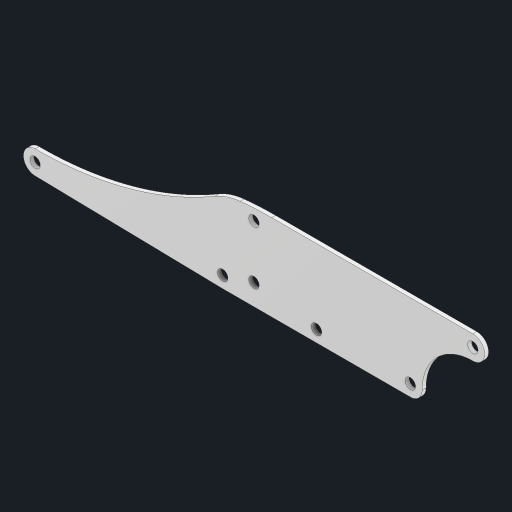
# Autodesk Inventor part: intake_base
Saved by Autodesk Inventor 2024 (Build 280153000, 153)
## iProperties
Created: 2023-08-21
Part Number: intake_base
Material: Acetal Resin, White
Document SubType Name: Modeling
Designer: Averey
Density: 1.425 g/cm^3
Appearance: Smooth - White
Author: Averey
Autodesk Inventor part; units mm, degrees
ref_plane "YZ Plane" through (0, 0, 0) normal (1, 0, 0) x (0, 1, 0)
ref_plane "XZ Plane" through (0, 0, 0) normal (0, 1, 0) x (-1, 0, 0)
ref_plane "XY Plane" through (0, 0, 0) normal (0, 0, 1) x (1, 0, 0)
sketch "Sketch1" plane through (0, 0, 0) normal (0, 0, 1) x (1, 0, 0)
  circle A0 centre (0, 0) radius 2.0955
  arc A1 (38.1, -4.7625) -> (41.4676, -3.3676) centre (38.1, 0) ccw
  circle A2 centre (-38.1, 0) radius 2.0955
  circle A3 centre (38.1, 0) radius 2.0955
  line L0 (-18.2636, 30.1625) -> (38.1, 30.1625)
  line L1 (38.1, -4.7625) -> (-38.1, -4.7625)
  arc A4 (-18.2636, 30.1625) -> (-31.0411, 29.5181) centre (-18.2636, -96.8375) ccw
  circle A5 centre (-114.3, 1.5875) radius 2.0955
  arc A6 (-115.6949, 6.1411) -> (-114.3992, -3.174) centre (-114.3, 1.5875) ccw
  arc A7 (-38.1992, -4.7615) -> (-38.1, -4.7625) centre (-38.1, 0) ccw
  line L2 (-38.1992, -4.7615) -> (-114.3992, -3.174)
  circle A8 centre (-25.4, 25.4) radius 2.0955
  circle A9 centre (63.5, 25.4) radius 2.0955
  arc A10 (66.8676, 22.0324) -> (63.5, 30.1625) centre (63.5, 25.4) ccw
  line L3 (38.1, 30.1625) -> (63.5, 30.1625)
  arc A11 (38.1, -4.7625) -> (42.8625, 0) centre (38.1, 0) ccw
  arc A12 (63.5, 20.6375) -> (63.5, 30.1625) centre (63.5, 25.4) ccw
  arc A13 (63.5, 20.6375) -> (42.8625, 0) centre (63.5, 0) ccw
  circle A14 centre (-25.4, 3.81) radius 2.0955
  arc A15 (-114.2961, 6.35) -> (-114.3992, -3.174) centre (-114.3, 1.5875) ccw
  arc A16 (-114.2961, 6.35) -> (-41.346, 26.1506) centre (-114.1779, 150.1975) ccw
  arc A17 (-31.0411, 29.5181) -> (-41.346, 26.1506) centre (-28.4856, 4.247) ccw
  point P0 (0, 0)
  point P1 (41.4676, -3.3676)
  dimension "d1" = 38.1
  dimension "d4" = 4.191
  dimension "d5" = 4.191
  dimension "d11" = 127
  dimension "d15" = 9.525
  dimension "d16" = 9.525
  dimension "d18" = 4.191
  dimension "d19" = 4.191
  dimension "d20" = 9.525
  dimension "d25" = 4.191
  dimension "d26" = 25.4
  constraints: 23 point on circle, 18 centre point, 8 coincident, 8 end point, 8 tangent, 1 horizontal, 1 horizontal alignment, 2 other
  measures "d1" distance of A1.centre A0.centre
  measures "d4" diameter of A3
  measures "d5" diameter of A0
  measures "d11" radius of A4
  measures "d15" diameter of A6
  measures "d16" diameter of A7
  measures "d18" diameter of A8
  measures "d19" diameter of A9
  measures "d20" diameter of A10
  measures "d25" diameter of A14
  measures "d26" radius of A17
extrude "Extrusion1" add sketch "Sketch1" along normal blind 1.5875
body "Solid1"
